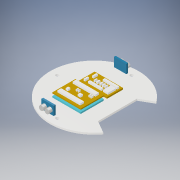
# Autodesk Inventor part: Top and middle round
Saved by Autodesk Inventor 2018 (Build 220112000, 112)
## iProperties
Created: 2018-10-22
Part Number: Top and middle round
Material: Generic
Document SubType Name: Modeling
Designer: Melda
Density: 1 g/cm^3
Appearance: White
Author: Melda
Autodesk Inventor part; units mm, degrees
ref_plane "YZ Plane" through (0, 0, 0) normal (1, 0, 0) x (0, 1, 0)
ref_plane "XZ Plane" through (0, 0, 0) normal (0, 1, 0) x (-1, 0, 0)
ref_plane "XY Plane" through (0, 0, 0) normal (0, 0, 1) x (1, 0, 0)
sketch "Sketch1" plane through (0, 0, 0) normal (0, 1, 0) x (-1, 0, 0)
  arc A0 (-99.8914, -75.1446) -> (-99.8914, 75.1446) centre (0, 0) ccw
  line L0 (-65, 0) -> (-65, 55)
  line L1 (-65, 55) -> (-99.8914, 75.1446)
  line L2 (-65, 0) -> (-65, -55)
  line L3 (-65, -55) -> (-99.8914, -75.1446)
  dimension "d0" = 250
  dimension "d4" = 55
  dimension "d6" = 120
  constraints: 8 end point, 2 point on circle, 1 centre point, 1 coincident, 1 vertical
  measures "d0" diameter of A0
  measures "d4" distance of L0.start L0.end
  measures "d6" angle of L1 L0
extrude "Extrusion1" add sketch "Sketch1" along normal blind 5
sketch "Sketch2" plane through (0, 5, 0) normal (0, 1, 0) x (1, 0, 0)
  circle A0 centre (-105, 0) radius 4
  circle A1 centre (0, 105) radius 4.3333
  circle A2 centre (0, -105) radius 4.3461
  arc A3 (99.8914, 75.1446) -> (99.8914, -75.1446) centre (0, 0) ccw
  dimension "d9" = 8
  dimension "d10" = 105
  dimension "d11" = 105
  dimension "d12" = 105
  constraints: 4 centre point, 2 point on circle
  measures "d9" diameter of A0
  measures "d10" distance of A3.centre A0.centre
  measures "d11" distance of A3.centre A1.centre
  measures "d12" distance of A3.centre A2.centre
extrude "Extrusion2" cut sketch "Sketch2" against normal blind 10
sketch "Sketch3" plane through (0, 5, 0) normal (0, 1, 0) x (1, 0, 0)
  line L0 (-57.0518, -61.5559) -> (22.9482, -61.5559)
  line L1 (22.9482, -61.5559) -> (22.9482, 3.4441)
  line L2 (22.9482, 3.4441) -> (-57.0518, 3.4441)
  line L3 (-57.0518, 3.4441) -> (-57.0518, -61.5559)
  line L4 (-57.0518, 12.7299) -> (22.9482, 12.7299)
  line L5 (22.9482, 12.7299) -> (22.9482, 57.7299)
  line L6 (22.9482, 57.7299) -> (-57.0518, 57.7299)
  line L7 (-57.0518, 57.7299) -> (-57.0518, 12.7299)
  point P0 (0, 0)
  dimension "d15" = 65
  dimension "d16" = 80
  dimension "d17" = 45
  constraints: 16 end point, 4 parallel, 2 horizontal, 2 perpendicular, 2 point on line
  measures "d15" distance of L2.end L0.start
  measures "d16" distance of L0.start L0.end
  measures "d17" distance of L6.end L4.start
extrude "Extrusion3" add sketch "Sketch3" along normal blind 4
sketch "Sketch4" plane through (0, 9, 0) normal (0, 1, 0) x (1, 0, 0)
  line L0 (-49.7839, -54.8102) -> (15.7968, -54.8102)
  line L1 (15.7968, -54.8102) -> (15.7968, -50.2626)
  line L2 (15.7968, -50.2626) -> (-49.7839, -50.2626)
  line L3 (-49.7839, -50.2626) -> (-49.7839, -54.8102)
  line L4 (-37.5773, -4.7869) -> (15.7968, -4.7869)
  line L5 (15.7968, -4.7869) -> (15.7968, 0)
  line L6 (15.7968, 0) -> (-37.5773, 0)
  line L7 (-37.5773, 0) -> (-37.5773, -4.7869)
  point P0 (0, 0)
  constraints: 16 end point, 4 parallel, 2 horizontal, 2 perpendicular, 1 point on line
extrude "Extrusion4" add sketch "Sketch4" along normal blind 6
sketch "Sketch5" plane through (0, 15, 0) normal (0, 1, 0) x (1, 0, 0)
  line L0 (-57.0518, -61.5559) -> (-57.0518, 3.4441) projected
  line L1 (22.9482, -61.5559) -> (22.9482, 3.4441) projected
  line L2 (-57.0518, -61.5559) -> (22.9482, -61.5559)
  line L3 (22.9482, -61.5559) -> (22.9482, 3.4441)
  line L4 (22.9482, 3.4441) -> (-57.0518, 3.4441)
  line L5 (-57.0518, 3.4441) -> (-57.0518, -61.5559)
  point P0 (0, 0)
  constraints: 8 end point, 2 parallel, 1 horizontal, 1 perpendicular
extrude "Extrusion5" add sketch "Sketch5" along normal blind 3
sketch "Sketch6" plane through (0, 18, 0) normal (0, 1, 0) x (1, 0, 0)
  line L0 (-49.7839, -50.2626) -> (-49.7839, -54.8102) projected
  line L1 (-49.7839, -54.8102) -> (14.6001, -54.8102)
  line L2 (14.6001, -54.8102) -> (14.6001, -44.279)
  line L3 (14.6001, -44.279) -> (-49.7839, -44.279)
  line L4 (-49.7839, -44.279) -> (-49.7839, -54.8102)
  line L5 (-49.7839, -11.7279) -> (14.6001, -11.7279)
  line L6 (14.6001, -11.7279) -> (14.6001, -1.6754)
  line L7 (14.6001, -1.6754) -> (-49.7839, -1.6754)
  line L8 (-49.7839, -1.6754) -> (-49.7839, -11.7279)
  line L9 (-43.8003, -37.338) -> (-37.5773, -37.338)
  line L10 (-37.5773, -37.338) -> (-37.5773, -30.1576)
  line L11 (-37.5773, -30.1576) -> (-43.8003, -30.1576)
  line L12 (-43.8003, -30.1576) -> (-43.8003, -37.338)
  line L13 (-26.8067, -25.8494) -> (-24.4133, -25.8494)
  line L14 (-24.4133, -25.8494) -> (-24.4133, -19.387)
  line L15 (-24.4133, -19.387) -> (-26.8067, -19.387)
  line L16 (-26.8067, -19.387) -> (-26.8067, -25.8494)
  line L17 (-21.3018, -25.8494) -> (-19.1477, -25.8494)
  line L18 (-19.1477, -25.8494) -> (-19.1477, -19.387)
  line L19 (-19.1477, -19.387) -> (-21.3018, -19.387)
  line L20 (-21.3018, -19.387) -> (-21.3018, -25.8494)
  line L21 (-12.2066, -35.4232) -> (-4.3082, -35.4232)
  line L22 (-4.3082, -35.4232) -> (-4.3082, -28.2428)
  line L23 (-4.3082, -28.2428) -> (-12.2066, -28.2428)
  line L24 (-12.2066, -28.2428) -> (-12.2066, -35.4232)
  line L25 (5.505, -22.6182) -> (8.3771, -22.6182)
  line L26 (8.3771, -22.6182) -> (8.3771, -15.7968)
  line L27 (8.3771, -15.7968) -> (5.505, -15.7968)
  line L28 (5.505, -15.7968) -> (5.505, -22.6182)
  line L29 (10.7706, -22.6182) -> (13.4034, -22.6182)
  line L30 (13.4034, -22.6182) -> (13.4034, -15.7968)
  line L31 (13.4034, -15.7968) -> (10.7706, -15.7968)
  line L32 (10.7706, -15.7968) -> (10.7706, -22.6182)
  point P0 (0, 0)
  constraints: 64 end point, 16 parallel, 8 horizontal, 8 perpendicular, 6 point on line
extrude "Extrusion6" add sketch "Sketch6" along normal blind 5
sketch "Sketch7" plane through (0, 9, 0) normal (0, 1, 0) x (1, 0, 0)
  line L0 (-50.502, 19.6264) -> (-45.9544, 19.6264)
  line L1 (-45.9544, 19.6264) -> (-45.9544, 30.8756)
  line L2 (-45.9544, 30.8756) -> (-50.502, 30.8756)
  line L3 (-50.502, 30.8756) -> (-50.502, 19.6264)
  line L4 (-45.9544, 39.0134) -> (-41.4068, 39.0134)
  line L5 (-41.4068, 39.0134) -> (-41.4068, 51.4594)
  line L6 (-41.4068, 51.4594) -> (-45.9544, 51.4594)
  line L7 (-45.9544, 51.4594) -> (-45.9544, 39.0134)
  line L8 (-37.8167, 19.6264) -> (0, 19.6264)
  line L9 (0, 19.6264) -> (0, 25.251)
  line L10 (0, 25.251) -> (-37.8167, 25.251)
  line L11 (-37.8167, 25.251) -> (-37.8167, 19.6264)
  line L12 (-33.2691, 30.8756) -> (-30.1576, 30.8756)
  line L13 (-30.1576, 30.8756) -> (-30.1576, 39.0134)
  line L14 (-30.1576, 39.0134) -> (-33.2691, 39.0134)
  line L15 (-33.2691, 39.0134) -> (-33.2691, 30.8756)
  line L16 (-26.0887, 30.8756) -> (-21.7805, 30.8756)
  line L17 (-21.7805, 30.8756) -> (-21.7805, 39.0134)
  line L18 (-21.7805, 39.0134) -> (-26.0887, 39.0134)
  line L19 (-26.0887, 39.0134) -> (-26.0887, 30.8756)
  line L20 (-17.2329, 30.8756) -> (-13.164, 30.8756)
  line L21 (-13.164, 30.8756) -> (-13.164, 39.0134)
  line L22 (-13.164, 39.0134) -> (-17.2329, 39.0134)
  line L23 (-17.2329, 39.0134) -> (-17.2329, 30.8756)
  line L24 (-9.5738, 30.8756) -> (-5.9836, 30.8756)
  line L25 (-5.9836, 30.8756) -> (-5.9836, 39.0134)
  line L26 (-5.9836, 39.0134) -> (-9.5738, 39.0134)
  line L27 (-9.5738, 39.0134) -> (-9.5738, 30.8756)
  line L28 (0, 30.8756) -> (-3.1115, 30.8756)
  line L29 (-3.1115, 30.8756) -> (-3.1115, 39.0134)
  line L30 (-3.1115, 39.0134) -> (0, 39.0134)
  line L31 (0, 39.0134) -> (0, 30.8756)
  line L32 (-21.7805, 45.2364) -> (18.9083, 45.2364)
  line L33 (18.9083, 45.2364) -> (18.9083, 51.4594)
  line L34 (18.9083, 51.4594) -> (-21.7805, 51.4594)
  line L35 (-21.7805, 51.4594) -> (-21.7805, 45.2364)
  line L36 (4.5476, 19.6264) -> (18.9083, 19.6264)
  line L37 (18.9083, 19.6264) -> (18.9083, 42.3642)
  line L38 (18.9083, 42.3642) -> (4.5476, 42.3642)
  line L39 (4.5476, 42.3642) -> (4.5476, 19.6264)
  point P0 (0, 0)
  constraints: 80 end point, 20 parallel, 17 point on line, 10 horizontal, 10 perpendicular
extrude "Extrusion7" add sketch "Sketch7" along normal blind 5
sketch "Sketch8" plane through (0, 5, 0) normal (0, 1, 0) x (1, 0, 0)
  line L0 (-45, -105) -> (-10, -105)
  line L1 (-10, -105) -> (-10, -100)
  line L2 (-10, -100) -> (-45, -100)
  line L3 (-45, -100) -> (-45, -105)
  line L4 (-159.3833, 0) -> (129.3404, 0)
  arc A0 (99.8914, 75.1446) -> (99.8914, -75.1446) centre (0, 0) ccw projected
  line L5 (-45, 105) -> (-10, 105)
  line L6 (-10, 105) -> (-10, 100)
  line L7 (-10, 100) -> (-45, 100)
  line L8 (-45, 100) -> (-45, 105)
  dimension "d28" = 5
  dimension "d29" = 35
  dimension "d31" = 100
  constraints: 18 end point, 4 symmetric about line, 2 horizontal, 2 parallel, 1 perpendicular
  measures "d28" distance of L2.end L0.start
  measures "d29" distance of L1.end L2.end
  measures "d31" distance from line of A0.centre L2
extrude "Extrusion8" add sketch "Sketch8" along normal blind 25
sketch "Sketch9" plane through (-10, 5, -105) normal (0, 0, -1) x (-1, 0, 0)
  circle A0 centre (9.692, 11.5) radius 6.5
  line L0 (-24.6001, 18) -> (39.7839, 18) projected
  circle A1 centre (25.415, 11.5004) radius 6.5
  point P0 (-10, -5)
  dimension "d34" = 13
  dimension "d35" = 13
  constraints: 2 centre point, 1 tangent
  measures "d34" diameter of A0
  measures "d35" diameter of A1
extrude "Extrusion9" add sketch "Sketch9" along normal blind 10
sketch "Sketch10" plane through (-45, 5, 105) normal (0, 0, 1) x (1, 0, 0)
  circle A0 centre (9.585, 11.5004) radius 6.5 projected
  circle A1 centre (9.585, 11.5004) radius 6.5
  circle A2 centre (25.308, 11.5) radius 6.5 projected
  circle A3 centre (25.308, 11.5) radius 6.5
  point P0 (45, -5)
  constraints: 2 centre point, 2 coincident
extrude "Extrusion10" add sketch "Sketch10" along normal blind 10
body "Solid1"
